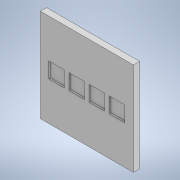
# Autodesk Inventor part: Base plana 4 cuadrados
Saved by Autodesk Inventor 2022.5 (Build 265521000, 521)
## iProperties
Created: 2023-09-27
Part Number: Base plana 4 cuadrados
Material: Genérico
Document SubType Name: Modeling
Designer: Carlos_Caucali
Density: 1 g/cm^3
Appearance: Valor por defecto
Author: Carlos_Caucali
Autodesk Inventor part; units mm, degrees
ref_plane "YZ Plane" through (0, 0, 0) normal (1, 0, 0) x (0, 1, 0)
ref_plane "XZ Plane" through (0, 0, 0) normal (0, 1, 0) x (-1, 0, 0)
ref_plane "XY Plane" through (0, 0, 0) normal (0, 0, 1) x (1, 0, 0)
sketch "Boceto1" plane through (0, 0, 0) normal (0, 0, 1) x (1, 0, 0)
  line L0 (-150, -150) -> (150, -150)
  line L1 (150, -150) -> (150, 150)
  line L2 (150, 150) -> (-150, 150)
  line L3 (-150, 150) -> (-150, -150)
  line L4 (-150, -150) -> (150, 150) construction
  line L5 (150, -150) -> (-150, 150) construction
  point P0 (0, 0)
  dimension "d0" = 300
  dimension "d1" = 300
  constraints: 12 end point, 2 midpoint, 2 parallel, 1 horizontal, 1 perpendicular
  measures "d0" distance of L2.end L1.end
  measures "d1" distance of L0.end L1.end
extrude "Extrusión1" add sketch "Boceto1" along normal blind 20
sketch "Boceto2" plane through (0, 0, 20) normal (0, 0, 1) x (1, 0, 0)
  line L0 (150, -150) -> (150, 150) construction
  line L1 (150, 150) -> (-150, 150) construction
  line L2 (-150, 150) -> (-150, -150) construction
  line L3 (-150, -150) -> (150, -150) construction
  line L4 (150, 150) -> (-150, 150) projected
  line L5 (0, 150) -> (0, -150)
  line L6 (-150, -150) -> (150, -150) projected
  line L7 (7.5, -25) -> (57.5, -25)
  line L8 (57.5, -25) -> (57.5, 25)
  line L9 (57.5, 25) -> (7.5, 25)
  line L10 (7.5, 25) -> (7.5, -25)
  line L11 (72.5, -25) -> (122.5, -25)
  line L12 (122.5, -25) -> (122.5, 25)
  line L13 (122.5, 25) -> (72.5, 25)
  line L14 (72.5, 25) -> (72.5, -25)
  line L15 (-7.5, -25) -> (-57.5, -25)
  line L16 (-57.5, -25) -> (-57.5, 25)
  line L17 (-57.5, 25) -> (-7.5, 25)
  line L18 (-7.5, 25) -> (-7.5, -25)
  line L19 (-72.5, -25) -> (-122.5, -25)
  line L20 (-122.5, -25) -> (-122.5, 25)
  line L21 (-122.5, 25) -> (-72.5, 25)
  line L22 (-72.5, 25) -> (-72.5, -25)
  point P0 (0, 0)
  point P1 (-85, -150)
  point P2 (215, -150)
  dimension "d4" = 50
  dimension "d5" = 50
  dimension "d6" = 15
  dimension "d7" = 125
  dimension "d10" = 65
  dimension "d15" = 300
  constraints: 34 end point, 8 symmetric about line, 2 horizontal, 2 midpoint, 2 parallel, 1 perpendicular, 10 other
  measures "d4" distance of L8.end L9.end
  measures "d5" distance of L7.end L8.end
  measures "d6" diameter of L10 L5
  measures "d7" distance between parallel lines of L9 L1
  measures "d10" distance of L7.start L11.start
  measures "d15" distance of L1.end L2.end
extrude "Extrusión2" cut sketch "Boceto2" against normal blind 5
equation "\"d7\" = -0.5 * d5 + 0.5 * d15"
equation "\"d10\" = d6 + d4"
